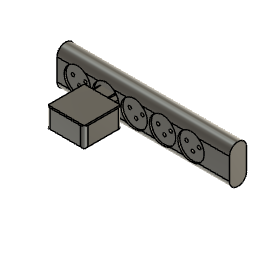
splitterv3 (Autodesk Fusion 360 design; units mm, degrees)
Autodesk Fusion 360 part; units mm, degrees
sketch "Sketch2" plane through (0, 0, 0) normal (0, 0, 1) x (1, 0, 0)
  line L0 (0, 0) -> (55.8, 0)
  line L1 (55.8, 0) -> (55.8, 55.8)
  line L2 (55.8, 55.8) -> (0, 55.8)
  line L3 (0, 55.8) -> (0, 0)
  dimension "d13" = 55.8
  dimension "d14" = 55.8
  constraint horizontal L0
  constraint vertical L1
  constraint horizontal L2
  constraint vertical L3
  constraint coincident L0.start L3.end
  measures "d13" distance of L0.start L0.end
  measures "d14" distance of L0.start L2.end
extrude "Extrude1" add sketch "Sketch2" along normal blind 29.64 makes body 1
sketch "Sketch6" plane through (0, 0, 0) normal (0, -1, 0) x (1, 0, 0)
  line L0 (0, 0) -> (55.8, 0)
  line L1 (55.8, 0) -> (55.8, 29.64)
  line L2 (55.8, 29.64) -> (0, 29.64)
  line L3 (0, 29.64) -> (0, 0)
  line L4 (0, 14.82) -> (34.62, 14.82) construction
  line L5 (0, 14.82) -> (0, 21.52) construction
  line L6 (0, 14.82) -> (6.1, 21.52)
  line L7 (0, 21.52) -> (6.1, 21.52) construction
  line L8 (0, 8.12) -> (6.1, 8.12) construction
  line L9 (0, 14.82) -> (6.1, 8.12)
  line L10 (6.1, 8.12) -> (28.52, 8.12)
  line L11 (6.1, 21.52) -> (28.52, 21.52)
  line L12 (28.52, 8.12) -> (34.62, 14.82)
  line L13 (27.28, 21.52) -> (34.62, 14.82)
  dimension "d18" = 34.62
  dimension "d19" = 6.7
  dimension "d20" = 6.1
  dimension "d21" = 13.4
  dimension "d22" = 21.18
  constraint midpoint L3 L4.start
  constraint perpendicular L3 L4
  constraint perpendicular L4 L5
  constraint perpendicular L5 L7
  constraint coincident L6.end L7.end
  constraint parallel L8 L10
  constraint parallel L6 L12
  constraint coincident L4.end L12.end
  constraint coincident L10.end L12.start
  constraint parallel L9 L13
  constraint coincident L11.end L13.start
  measures "d18" distance of L4.start L4.end
  measures "d19" distance of L4.start L5.end
  measures "d20" distance of L5.end L6.end
extrude "Extrude2" add sketch "Sketch6" along normal blind 18.58 contours L6 L9 L10 L11 L12 L13 bodies 1
sketch "Sketch7" plane through (0, -18.58, 0) normal (0, -1, 0) x (1, 0, 0)
  line L0 (0, 14.82) -> (6.1, 8.12)
  line L1 (6.1, 8.12) -> (28.52, 8.12)
  line L2 (28.52, 8.12) -> (34.62, 14.82)
  line L3 (34.62, 14.82) -> (27.28, 21.52)
  line L4 (27.28, 21.52) -> (6.1, 21.52)
  line L5 (6.1, 21.52) -> (0, 14.82)
  line L6 (0, 14.82) -> (8.08, 14.82) construction
  circle A0 centre (8.08, 14.82) radius 1.98
  line L7 (34.62, 14.82) -> (26.54, 14.82) construction
  circle A1 centre (26.54, 14.82) radius 1.98
  dimension "d26" = 8.08
  dimension "d27" = 3.96
  dimension "d29" = 3.96
  constraint coincident L0.start L5.end
  constraint horizontal L6
  constraint coincident L6.end A0.centre
  constraint coincident L2.end L3.start
  constraint coincident L7.end A1.centre
  constraint equal L6 L7
  constraint parallel L6 L7
  measures "d26" distance of L0.start L6.end
  measures "d27" diameter of A0
  measures "d29" diameter of A1
extrude "Extrude3" add sketch "Sketch7" along normal blind 17.29 contours A0 | A1 bodies 1
fillet "Fillet1" radius 1.98 1 faces at (7.9462, -35.87, 14.2631) on bodies 1
fillet "Fillet2" radius 1.98 1 faces at (26.2989, -35.87, 15.4344) on bodies 1
fillet "Fillet3" radius 2 6 edges at (34.62, -9.29, 14.82) (27.28, -9.29, 21.52) (6.1, -9.29, 21.52) (28.52, -9.29, 8.12) (6.1, -9.29, 8.12) (0, -9.29, 14.82) on bodies 1
chamfer "Chamfer1" distance 1.25 angle 45 8 edges at (55.8, 27.9, 0) (27.9, 0, 0) (0, 27.9, 0) (27.9, 55.8, 0) (27.9, 0, 29.64) (55.8, 27.9, 29.64) (27.9, 55.8, 29.64) (0, 27.9, 29.64) on bodies 1
fillet "Fillet4" radius 5.5 4 edges at (55.8, 0, 14.82) (55.8, 55.8, 14.82) (0, 0, 14.82) (0, 55.8, 14.82) on bodies 1
copy_body "Body->Comp1" bodies 1 removing the originals makes body 2 in component "Charger"
sketch "Sketch1" plane through (0, 0, 0) normal (0, 1, 0) x (1, 0, 0) in component "Splitter"
  line L0 (0, 0) -> (254.1, 0)
  line L1 (254.1, 0) -> (254.1, -57.2)
  line L2 (254.1, -57.2) -> (0, -57.2)
  line L3 (0, -57.2) -> (0, 0)
  line L4 (0, -28.6) -> (29.9, -28.6) construction
  circle A0 centre (29.9, -28.6) radius 19.4
  line L5 (29.9, -28.6) -> (71.78, -28.6) construction
  circle A1 centre (71.78, -28.6) radius 19.4
  line L6 (71.78, -28.6) -> (113.66, -28.6) construction
  circle A2 centre (113.66, -28.6) radius 19.4
  line L7 (113.66, -28.6) -> (155.54, -28.6) construction
  circle A3 centre (155.54, -28.6) radius 19.4
  line L8 (155.54, -28.6) -> (197.42, -28.6) construction
  circle A4 centre (197.42, -28.6) radius 19.4
  circle A5 centre (20.675, -30.7855) radius 2.425
  circle A6 centre (39.125, -30.7855) radius 2.425
  circle A7 centre (29.9, -21.555) radius 2.425
  line L9 (20.675, -30.7855) -> (39.125, -30.7855) construction
  line L10 (20.675, -30.7855) -> (29.9, -21.555) construction
  line L11 (39.125, -30.7855) -> (29.9, -21.555) construction
  line L12 (29.9, -21.555) -> (29.9, -48) construction
  line L13 (20.675, -30.7855) -> (10.6235, -30.7855) construction
  line L14 (39.125, -30.7855) -> (49.1765, -30.7855) construction
  line L15 (20.675, -30.7855) -> (62.555, -30.7855) construction
  line L16 (62.555, -30.7855) -> (104.435, -30.7855) construction
  line L17 (104.435, -30.7855) -> (146.315, -30.7855) construction
  line L18 (146.315, -30.7855) -> (188.195, -30.7855) construction
  circle A8 centre (146.315, -30.7855) radius 2.425
  circle A9 centre (188.195, -30.7855) radius 2.425
  circle A10 centre (104.435, -30.7855) radius 2.425
  circle A11 centre (62.555, -30.7855) radius 2.425
  line L19 (29.9, -21.555) -> (71.78, -21.555) construction
  circle A12 centre (71.78, -21.555) radius 2.425
  line L20 (71.78, -21.555) -> (113.66, -21.555) construction
  circle A13 centre (113.66, -21.555) radius 2.425
  line L21 (113.66, -21.555) -> (155.54, -21.555) construction
  circle A14 centre (155.54, -21.555) radius 2.425
  line L22 (155.54, -21.555) -> (197.42, -21.555) construction
  circle A15 centre (197.42, -21.555) radius 2.425
  line L23 (71.78, -21.555) -> (81.005, -30.7855) construction
  circle A16 centre (81.005, -30.7855) radius 2.425
  line L24 (113.66, -21.555) -> (122.885, -30.7855) construction
  circle A17 centre (122.885, -30.7855) radius 2.425
  line L25 (155.54, -21.555) -> (164.765, -30.7855) construction
  circle A18 centre (164.765, -30.7855) radius 2.425
  line L26 (197.42, -21.555) -> (206.645, -30.7855) construction
  circle A19 centre (206.645, -30.7855) radius 2.425
  dimension "d51" = 254.1
  dimension "d52" = 57.2
  dimension "d54" = 29.9
  dimension "d55" = 38.8
  dimension "d59" = 41.88
  dimension "d60" = 38.8
  dimension "d61" = 38.8
  dimension "d62" = 38.8
  dimension "d63" = 38.8
  dimension "d65" = 4.85
  dimension "d66" = 4.85
  dimension "d67" = 4.85
  dimension "d68" = 18.45
  dimension "d69" = 13.05
  dimension "d70" = 13.05
  dimension "d73" = 26.445
  dimension "d75" = 41.88
  dimension "d78" = 4.85
  dimension "d79" = 4.85
  dimension "d80" = 4.85
  dimension "d81" = 4.85
  dimension "d82" = 41.88
  dimension "d83" = 4.85
  dimension "d84" = 41.88
  dimension "d85" = 4.85
  dimension "d86" = 41.88
  dimension "d87" = 4.85
  dimension "d88" = 41.88
  dimension "d89" = 4.85
  dimension "d90" = 4.85
  dimension "d91" = 4.85
  dimension "d92" = 4.85
  dimension "d93" = 4.85
  constraint horizontal L0
  constraint vertical L1
  constraint horizontal L2
  constraint vertical L3
  constraint coincident L0.start L3.end
  constraint midpoint L3 L4.start
  constraint perpendicular L3 L4
  constraint coincident L4.end A0.centre
  constraint parallel L4 L5
  constraint coincident L5.end A1.centre
  constraint parallel L5 L6
  constraint equal L5 L6
  constraint coincident L6.end A2.centre
  constraint parallel L6 L7
  constraint equal L6 L7
  constraint coincident L7.end A3.centre
  constraint parallel L7 L8
  constraint equal L7 L8
  constraint coincident L8.end A4.centre
  constraint coincident A5.centre L9.start
  constraint horizontal L9
  constraint coincident A6.centre L9.end
  constraint coincident A7.centre L10.end
  constraint coincident A0 L12.end
  constraint vertical L12
  constraint coincident A0 L13.end
  constraint horizontal L13
  constraint horizontal L14
  constraint coincident A0 L14.end
  constraint equal L13 L14
  constraint parallel L14 L15
  constraint parallel L15 L16
  constraint equal L15 L16
  constraint parallel L16 L17
  constraint equal L16 L17
  constraint parallel L17 L18
  constraint equal L17 L18
  constraint coincident L17.end L18.start
  constraint coincident L18.end A9.centre
  constraint coincident L16.end L17.start
  constraint coincident L15.end L16.start
  constraint perpendicular L12 L19
  constraint coincident L19.end A12.centre
  constraint parallel L19 L20
  constraint coincident L20.end A13.centre
  constraint parallel L20 L21
  constraint coincident L21.end A14.centre
  constraint parallel L21 L22
  constraint coincident L22.end A15.centre
  constraint parallel L11 L23
  constraint equal L11 L23
  constraint coincident L23.end A16.centre
  constraint parallel L23 L24
  constraint equal L23 L24
  constraint coincident L24.end A17.centre
  constraint parallel L24 L25
  constraint equal L24 L25
  constraint coincident L25.end A18.centre
  constraint equal L25 L26
  constraint parallel L25 L26
  constraint coincident L26.end A19.centre
  measures "d51" distance of L0.start L0.end
  measures "d52" distance of L0.start L2.end
  measures "d54" distance of L4.start L4.end
  measures "d55" diameter of A0
  measures "d59" distance of L4.end L5.end
  measures "d60" diameter of A1
  measures "d61" diameter of A2
  measures "d62" diameter of A3
  measures "d63" diameter of A4
  measures "d65" diameter of A5
  measures "d66" diameter of A6
  measures "d67" diameter of A7
  measures "d68" distance of A5.centre A6.centre
  measures "d69" distance of A5.centre A7.centre
  measures "d70" distance of A6.centre A7.centre
  measures "d73" distance of A7.centre L12.end
  measures "d75" distance of A5.centre L15.end
  measures "d78" diameter of A8
  measures "d79" diameter of A9
  measures "d80" diameter of A10
  measures "d81" diameter of A11
  measures "d82" distance of A7.centre L19.end
  measures "d83" diameter of A12
  measures "d84" distance of L19.end L20.end
  measures "d85" diameter of A13
  measures "d86" distance of L20.end L21.end
  measures "d87" diameter of A14
  measures "d88" distance of L21.end L22.end
  measures "d89" diameter of A15
  measures "d90" diameter of A16
  measures "d91" diameter of A17
  measures "d92" diameter of A18
  measures "d93" diameter of A19
sketch "Sketch3" plane through (0, 0, 0) normal (0, 1, 0) x (1, 0, 0) in component "Splitter"
  line L0 (0, 0) -> (254.1, 0)
  line L1 (254.1, 0) -> (254.1, -57.2)
  line L2 (254.1, -57.2) -> (0, -57.2)
  line L3 (0, -57.2) -> (0, 0)
  dimension "d94" = 254.1
  dimension "d95" = 57.2
  constraint horizontal L0
  constraint vertical L1
  constraint horizontal L2
  constraint vertical L3
  constraint coincident L0.start L3.end
  measures "d94" distance of L0.start L0.end
  measures "d95" distance of L0.start L2.end
extrude "Extrude1'" add sketch "Sketch3" along normal blind 25.25 separate body makes body 3 in component "Splitter"
extrude "Extrude2'" cut sketch "Sketch1" along normal blind 2.8 contours A0 | A1 | A2 | A3 | A4 bodies 3 in component "Splitter"
extrude "Extrude3'" cut 15 faces at (20.2642, 0, 29.9974) (39.8974, 0, 30.3223) (29.3804, 0, 19.8198) (63.2993, 0, 31.4355) (79.1092, 0, 30.5828) (69.8842, 0, 21.3524) (106.3308, 0, 30.5828) (120.9892, 0, 30.5828) (111.7642, 0, 21.3524) (147.1747, 0, 31.4711) (163.1286, 0, 31.0682) (156.065, 0, 20.855) (186.5586, 0, 31.0682) (205.0086, 0, 31.0682) (196.895, 0, 22.255) along direction (0, 1, 0) blind 19.5 on bodies 3 bodies 3 in component "Splitter"
fillet "Fillet1'" radius 12.625 4 edges at (127.05, 0, 57.2) (127.05, 25.25, 57.2) (127.05, 0, 0) (127.05, 25.25, 0) on bodies 3 in component "Splitter"
move_body "Move1" bodies 2 to x (-1, 0, 0) y (0, -1, 0) z (0, 0, 1) at (55.8, 55.8, 0) in component "Charger"
move_body "Move2" bodies 2 to x (-1, 0, 0) y (0, 1, 0) z (0, 0, -1) at (55.8, 0, 59.28) in component "Charger"
component "Charger" placed x (1, 0, 0) y (0, 1, 0) z (0, 0, 1) at (54.465, -70.19, -13.6745)
component "Splitter" placed x (1, 0, 0) y (0, 1, 0) z (0, 0, 1) at (0, 0, 0)
equation "charger_main_wid = 55.8 mm"
equation "charger_main_height = 55.8 mm"
equation "charger_socket_height = 18.58 mm"
equation "charger_main_dep = 29.64 mm"
equation "charger_prong_rad = 1.98 mm"
equation "charger_socket_wid = 34.62 mm"
equation "charger_socket_dep = 13.4 mm"
equation "d13 = charger_main_wid"
equation "d14 = charger_main_height"
equation "d15 = charger_main_dep"
equation "charger_between_prongs = 14.5 mm"
equation "d18 = charger_socket_wid"
equation "d19 = charger_socket_dep / 2"
equation "d20 = ( charger_socket_wid - charger_between_prongs - 4 * charger_prong_rad ) / 2"
equation "d21 = charger_socket_dep"
equation "d23 = -charger_socket_dep"
equation "d24 = charger_socket_height"
equation "d26 = ( charger_socket_wid - charger_between_prongs - 4 * charger_prong_rad ) / 2 + charger_prong_rad"
equation "d27 = charger_prong_rad * 2"
equation "d29 = charger_prong_rad * 2"
equation "charger_prong_height = 19.27 mm"
equation "d31 = charger_prong_height - charger_prong_rad"
equation "d34 = charger_prong_rad"
equation "d36 = charger_prong_rad"
equation "splitter_height = 57.2 mm"
equation "splitter_wid = 254.1 mm"
equation "splitter_dep = 25.25 mm"
equation "splitter_socket_diam = 38.8 mm"
equation "splitter_socket_dep = 2.8 mm"
equation "splitter_bet_main_prong_edges = 13.6 mm"
equation "splitter_bet_sec_prong_edges = 8.2 mm"
equation "splitter_prong_dep = 19.5 mm"
equation "splitter_bet_sockets = 3.08 mm"
equation "d51 = splitter_wid"
equation "d52 = splitter_height"
equation "splitter_first_socket = 10.5 mm"
equation "d54 = splitter_first_socket + splitter_socket_diam / 2"
equation "d55 = splitter_socket_diam"
equation "d59 = splitter_socket_diam + splitter_bet_sockets"
equation "d60 = splitter_socket_diam"
equation "d61 = splitter_socket_diam"
equation "d62 = splitter_socket_diam"
equation "d63 = splitter_socket_diam"
equation "splitter_prong_diam = 4.85 mm"
equation "d65 = splitter_prong_diam"
equation "d66 = splitter_prong_diam"
equation "d67 = splitter_prong_diam"
equation "d68 = splitter_bet_main_prong_edges + splitter_prong_diam"
equation "d69 = splitter_bet_sec_prong_edges + splitter_prong_diam"
equation "d70 = splitter_bet_sec_prong_edges + splitter_prong_diam"
equation "splitter_bottom_prong_to_furthest_edge = 28.87 mm"
equation "d73 = splitter_bottom_prong_to_furthest_edge - splitter_prong_diam / 2"
equation "d75 = splitter_socket_diam + splitter_bet_sockets"
equation "d78 = splitter_prong_diam"
equation "d79 = splitter_prong_diam"
equation "d80 = splitter_prong_diam"
equation "d81 = splitter_prong_diam"
equation "d82 = splitter_socket_diam + splitter_bet_sockets"
equation "d83 = splitter_prong_diam"
equation "d84 = splitter_socket_diam + splitter_bet_sockets"
equation "d85 = splitter_prong_diam"
equation "d86 = splitter_socket_diam + splitter_bet_sockets"
equation "d87 = splitter_prong_diam"
equation "d88 = splitter_socket_diam + splitter_bet_sockets"
equation "d89 = splitter_prong_diam"
equation "d90 = splitter_prong_diam"
equation "d91 = splitter_prong_diam"
equation "d92 = splitter_prong_diam"
equation "d93 = splitter_prong_diam"
equation "d94 = splitter_wid"
equation "d95 = splitter_height"
equation "d96 = splitter_dep"
equation "d98 = splitter_socket_dep"
equation "d100 = -splitter_prong_dep"
equation "d103 = splitter_dep / 2"
